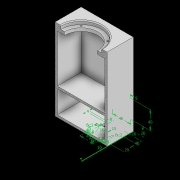
# Autodesk Inventor part: groovev2
Saved by Autodesk Inventor 2022 (Build 260153000, 153)
## iProperties
Created: 2022-06-28
Part Number: groovev2
Material: Generic
Document SubType Name: Modeling
Designer: Fuzzyfish
Density: 1 g/cm^3
Appearance: Default
Author: Fuzzyfish
Autodesk Inventor part; units mm, degrees
ref_plane "YZ Plane" through (0, 0, 0) normal (1, 0, 0) x (0, 1, 0)
ref_plane "XZ Plane" through (0, 0, 0) normal (0, 1, 0) x (-1, 0, 0)
sketch "Sketch1" plane through (0, 0, 0) normal (0, 1, 0) x (-1, 0, 0)
  line L0 (0, 0) -> (105, 0)
  line L1 (105, 0) -> (105, -105)
  line L2 (105, -105) -> (0, -105)
  line L3 (0, -105) -> (0, 0)
  circle A0 centre (52.5, -52.5) radius 36.5
  dimension "d0" = 105
  dimension "d1" = 105
  dimension "d2" = 52.5
  dimension "d3" = 52.5
  dimension "d4" = 73
  constraints: 8 end point, 2 parallel, 1 centre point, 1 horizontal, 1 perpendicular
  measures "d0" distance of L0.end L1.end
  measures "d1" distance of L1.end L2.end
  measures "d2" distance from line of L1 A0.centre
  measures "d3" distance from line of L0 A0.centre
  measures "d4" diameter of A0
extrude "Extrusion1" add sketch "Sketch1" along normal blind 7
sketch "Sketch3" plane through (-105, 0, 0) normal (0, 0, 1) x (1, 0, 0)
  line L0 (105, 7) -> (0, 7) projected
  line L1 (0, 7) -> (105, 7)
  line L2 (105, 7) -> (105, -105)
  line L3 (105, -105) -> (0, -105)
  line L4 (0, -105) -> (0, 7)
  line L5 (0, 0) -> (105, 0) projected
  dimension "d7" = 105
  constraints: 8 end point, 2 parallel, 1 horizontal, 1 perpendicular
  measures "d7" distance between parallel lines of L5 L3
extrude "Extrusion2" add sketch "Sketch3" along normal blind 5
sketch "Sketch4" plane through (-105, 0, -105) normal (-1, 0, 0) x (0, 0, 1)
  line L0 (0, 0) -> (0, 7) projected
  line L1 (0, 7) -> (110, 7)
  line L2 (110, 7) -> (110, -105)
  line L3 (110, -105) -> (0, -105)
  line L4 (0, -105) -> (0, 7)
  point P0 (105, 0)
  constraints: 8 end point, 2 parallel, 1 horizontal, 1 perpendicular
extrude "Extrusion3" add sketch "Sketch4" along normal blind 5
sketch "Sketch6" plane through (0, 0, -105) normal (0, 0, -1) x (-1, 0, 0)
  line L0 (0, 7) -> (110, 7) projected
  line L1 (110, -105) -> (110, 7) projected
  line L2 (0, 7) -> (110, 7)
  line L3 (110, 7) -> (110, -105)
  line L4 (110, -105) -> (0, -105)
  line L5 (0, -105) -> (0, 7)
  point P0 (0, 0)
  constraints: 8 end point, 2 parallel, 1 horizontal, 1 perpendicular
extrude "Extrusion4" add sketch "Sketch6" along normal blind 5
sketch "Sketch7" plane through (0, -105, 0) normal (1, 0, 0) x (0, 0, -1)
  line L0 (-5, 0) -> (-5, 112) projected
  line L1 (105, 0) -> (110, 0) projected
  line L2 (-5, 112) -> (110, 112)
  line L3 (110, 112) -> (110, 0)
  line L4 (110, 0) -> (-5, 0)
  line L5 (-5, 0) -> (-5, 112)
  point P0 (0, 105)
  constraints: 8 end point, 2 parallel, 1 horizontal, 1 perpendicular
extrude "Extrusion5" add sketch "Sketch7" along normal blind 5
sketch "Sketch8" plane through (-110, -105, -110) normal (0, -1, 0) x (1, 0, 0)
  line L0 (0, 115) -> (115, 115) projected
  line L1 (0, 0) -> (115, 0) projected
  line L2 (0, 115) -> (115, 115)
  line L3 (115, 115) -> (115, 0)
  line L4 (115, 0) -> (0, 0)
  line L5 (0, 0) -> (0, 115)
  point P0 (110, 110)
  constraints: 8 end point, 2 parallel, 1 horizontal, 1 perpendicular
extrude "Extrusion6" add sketch "Sketch8" along normal blind 5
sketch "Sketch9" plane through (0, 7, 0) normal (0, 1, 0) x (1, 0, 0)
  line L0 (-110, -5) -> (-110, 110) projected
  line L1 (-110, -5) -> (5, -5) projected
  line L2 (5, 110) -> (5, -5) projected
  line L3 (-110, 110) -> (5, 110) projected
  circle A0 centre (-52.5, 52.5) radius 36.5 projected
  line L4 (-110, -5) -> (-110, 110) projected
  line L5 (-110, 110) -> (5, 110) projected
  line L6 (-110, -5) -> (5, -5)
  line L7 (5, -5) -> (5, 110)
  line L8 (5, 110) -> (-110, 110)
  line L9 (-110, 110) -> (-110, -5)
  circle A1 centre (-52.5, 52.5) radius 45
  dimension "d18" = 90
  constraints: 8 end point, 2 parallel, 1 centre point, 1 coincident, 1 horizontal, 1 perpendicular
  measures "d18" diameter of A1
extrude "Extrusion7" add sketch "Sketch9" along normal blind 8 contours L0 L3 L2 L1
sketch "Sketch10" plane through (-52.5, 7, -52.5) normal (0, 1, 0) x (1, 0, 0)
  line L0 (57.5, -57.5) -> (-57.5, -57.5) construction
  line L1 (57.5, 57.5) -> (57.5, -57.5) construction
  line L2 (-57.5, -57.5) -> (57.5, 57.5) construction
  line L3 (57.5, 57.5) -> (-57.5, 57.5) construction
  line L4 (-57.5, 57.5) -> (57.5, -57.5) construction
  circle A0 centre (0, 0) radius 41.75 construction
  circle A1 centre (-29.5217, -29.5217) radius 1.9
  circle A2 centre (-29.5217, 29.5217) radius 1.9
  circle A3 centre (29.5217, 29.5217) radius 1.9
  circle A4 centre (29.5217, -29.5217) radius 1.9
  line L5 (0, -57.5) -> (0, 57.5) construction
  point P0 (52.5, -52.5)
  dimension "d21" = 3.8
  dimension "d22" = 83.5
  dimension "d23" = 3.8
  dimension "d24" = 3.8
  dimension "d25" = 3.8
  dimension "d26" = 45
  constraints: 8 end point, 5 centre point, 4 point on circle, 4 point on line, 3 midpoint, 2 perpendicular
  measures "d21" diameter of A1
  measures "d22" diameter of A0
  measures "d23" diameter of A2
  measures "d24" diameter of A3
  measures "d25" diameter of A4
  measures "d26" angle of L5 L2
extrude "Extrusion8" cut sketch "Sketch10" against normal blind 5
ref_plane "Work Plane1" through (0, 0, -52.5) normal (0, 0, -1) x (-1, 0, 0)
split "Split2" [suppressed]
chamfer "Chamfer1" distance 2 angle 45 1 edges at (-97.5, 15, -52.5)
sketch "Sketch15" plane through (0, 0, -52.5) normal (0, 0, -1) x (-1, 0, 0)
  line L0 (105, 14) -> (99.9142, 14)
  line L1 (99.9142, 14) -> (98.5, 12.5858)
  line L2 (98.5, 12.5858) -> (98.5, 6)
  line L3 (98.5, 6) -> (90, 6)
  line L4 (90, 6) -> (90, 1)
  line L5 (90, 1) -> (100, 1)
  arc A0 (106, -5) -> (100, 1) centre (100, -5) ccw
  line L6 (106, -5) -> (106, -100)
  arc A1 (100, -106) -> (106, -100) centre (100, -100) ccw
  line L7 (100, -106) -> (5, -106)
  arc A2 (-1, -100) -> (5, -106) centre (5, -100) ccw
  line L8 (-1, -100) -> (-1, -5)
  arc A3 (5, 1) -> (-1, -5) centre (5, -5) ccw
  line L9 (5, 1) -> (15, 1)
  line L10 (15, 1) -> (15, 6)
  line L11 (15, 6) -> (6.5, 6)
  line L12 (6.5, 6) -> (6.5, 12.5858)
  line L13 (6.5, 12.5858) -> (5.0858, 14)
  line L14 (5.0858, 14) -> (0, 14)
  arc A4 (0, 14) -> (-4, 10) centre (0, 10) ccw
  line L15 (-4, 10) -> (-4, -105)
  arc A5 (-4, -105) -> (0, -109) centre (0, -105) ccw
  line L16 (0, -109) -> (105, -109)
  arc A6 (105, -109) -> (109, -105) centre (105, -105) ccw
  line L17 (109, -105) -> (109, 10)
  arc A7 (109, 10) -> (105, 14) centre (105, 10) ccw
  line L18 (89, 0) -> (89, 7) projected
  line L19 (89, 7) -> (97.5, 7) projected
  line L20 (97.5, 7) -> (97.5, 13) projected
  line L21 (97.5, 13) -> (99.5, 15) projected
  line L22 (99.5, 15) -> (110, 15) projected
  line L23 (110, 15) -> (110, -110) projected
  line L24 (110, -110) -> (-5, -110) projected
  line L25 (-5, -110) -> (-5, 15) projected
  line L26 (-5, 15) -> (5.5, 15) projected
  line L27 (5.5, 15) -> (7.5, 13) projected
  line L28 (7.5, 13) -> (7.5, 7) projected
  line L29 (7.5, 7) -> (16, 7) projected
  line L30 (16, 7) -> (16, 0) projected
  line L31 (16, 0) -> (0, 0) projected
  line L32 (0, 0) -> (0, -105) projected
  line L33 (0, -105) -> (105, -105) projected
  line L34 (105, -105) -> (105, 0) projected
  line L35 (105, 0) -> (89, 0) projected
  constraints: 36 end point, 16 point on circle, 8 centre point
extrude "Extrusion11" [suppressed]
sketch "Sketch16" plane through (-110, -110, -110) normal (0, -1, 0) x (1, 0, 0)
  line L0 (10, 57.5) -> (105, 57.5) projected
  line L1 (10, 57.5) -> (10, 54.5) projected
  line L2 (10, 54.5) -> (105, 54.5) projected
  line L3 (105, 57.5) -> (105, 54.5) projected
  circle A0 centre (57.5, 56) radius 2
  line L4 (115, 57.5) -> (0, 57.5) projected
  point P0 (110, 110)
  point P1 (110, 57.5)
  point P2 (5, 57.5)
  dimension "d53" = 95
  dimension "d54" = 47.5
  dimension "d55" = 4
  dimension "d58" = 1.5
  constraints: 1 centre point
  measures "d53" distance of L1.end L2.end
  measures "d54" distance from line of L1 A0.centre
  measures "d55" diameter of A0
  measures "d58" distance from line of L0 A0.centre
extrude "Extrusion14" [suppressed]
sketch "Sketch17" plane through (0, 0, -110) normal (0, 0, -1) x (-1, 0, 0)
  line L0 (110, 15) -> (110, -110) projected
  line L1 (110, -110) -> (-5, -110)
  line L2 (-5, -110) -> (-5, -160)
  line L3 (-5, -160) -> (110, -160)
  line L4 (110, -160) -> (110, -110)
  line L5 (-5, 15) -> (-5, -110) projected
  point P0 (0, 0)
  dimension "d59" = 50
  constraints: 8 end point, 2 parallel, 1 collinear, 1 horizontal, 1 perpendicular
  measures "d59" distance between parallel lines of L1 L3
extrude "Extrusion15" add sketch "Sketch17" against normal blind 5
sketch "Sketch18" plane through (5, -105, 0) normal (1, 0, 0) x (0, 0, -1)
  line L0 (105, -5) -> (-5, -5)
  line L1 (-5, -5) -> (-5, -55)
  line L2 (-5, -55) -> (105, -55)
  line L3 (105, -55) -> (105, -5)
  line L4 (-5, -5) -> (-5, 120) projected
  line L5 (110, -55) -> (105, -55) projected
  point P0 (0, 105)
  constraints: 8 end point, 2 collinear, 2 parallel, 1 horizontal, 1 perpendicular
extrude "Extrusion16" add sketch "Sketch18" against normal blind 5
sketch "Sketch19" plane through (-105, 0, 5) normal (0, 0, 1) x (1, 0, 0)
  line L0 (105, -110) -> (-5, -110) projected
  line L1 (-5, -160) -> (105, -160) projected
  line L2 (-5, -110) -> (105, -110)
  line L3 (105, -110) -> (105, -160)
  line L4 (105, -160) -> (-5, -160)
  line L5 (-5, -160) -> (-5, -110)
  point P0 (105, 0)
  constraints: 8 end point, 2 parallel, 1 horizontal, 1 perpendicular
extrude "Extrusion17" add sketch "Sketch19" against normal blind 5
sketch "Sketch20" plane through (-110, 0, -105) normal (-1, 0, 0) x (0, 0, 1)
  line L0 (-5, -160) -> (110, -160) projected
  line L1 (0, -110) -> (105, -110)
  line L2 (105, -110) -> (105, -160)
  line L3 (105, -160) -> (0, -160)
  line L4 (0, -160) -> (0, -110)
  point P0 (105, 0)
  constraints: 8 end point, 2 parallel, 1 horizontal, 1 perpendicular, 1 point on line
extrude "Extrusion18" add sketch "Sketch20" against normal blind 5
sketch "Sketch21" plane through (-110, -160, -110) normal (0, -1, 0) x (1, 0, 0)
  line L0 (115, 0) -> (0, 0) projected
  line L1 (115, 115) -> (0, 115) projected
  line L2 (0, 0) -> (115, 0)
  line L3 (115, 0) -> (115, 115)
  line L4 (115, 115) -> (0, 115)
  line L5 (0, 115) -> (0, 0)
  point P0 (110, 110)
  constraints: 8 end point, 2 parallel, 1 horizontal, 1 perpendicular
extrude "Extrusion19" add sketch "Sketch21" along normal blind 5
sketch "Sketch25" plane through (-110, -165, -110) normal (0, -1, 0) x (1, 0, 0)
  line L0 (65, 50) -> (105, 50) construction
  line L1 (105, 50) -> (105, 10) construction
  line L2 (105, 10) -> (65, 10) construction
  line L3 (65, 10) -> (65, 50) construction
  line L4 (65, 50) -> (105, 10) construction
  line L5 (105, 50) -> (65, 10) construction
  circle A0 centre (67, 46) radius 1.9
  circle A1 centre (103, 46) radius 1.9
  circle A2 centre (67, 25) radius 1.9
  circle A3 centre (103, 21) radius 1.9
  circle A4 centre (103, 46) radius 3.9
  circle A5 centre (67, 25) radius 3.9
  circle A6 centre (103, 21) radius 3.9
  line L6 (115, 0) -> (115, 115) projected
  line L7 (0, 0) -> (115, 0) projected
  line L8 (83, 14) -> (73, 14)
  line L9 (73, 14) -> (73, 29)
  line L10 (73, 29) -> (83, 29)
  line L11 (83, 29) -> (83, 14)
  line L12 (63, 50) -> (71, 50)
  line L13 (71, 50) -> (71, 42)
  line L14 (71, 42) -> (63, 42)
  line L15 (63, 42) -> (63, 50)
  line L16 (63, 50) -> (71, 42) construction
  line L17 (71, 50) -> (63, 42) construction
  point P0 (110, 110)
  point P1 (85, 30)
  dimension "d101" = 40
  dimension "d102" = 40
  dimension "d103" = 3.8
  dimension "d104" = 3.8
  dimension "d105" = 3.8
  dimension "d106" = 3.8
  dimension "d107" = 4
  dimension "d108" = 2
  dimension "d109" = 2
  dimension "d110" = 4
  dimension "d111" = 25
  dimension "d112" = 2
  dimension "d113" = 29
  dimension "d114" = 2
  dimension "d116" = 2
  dimension "d117" = 2
  dimension "d118" = 2
  dimension "d124" = 10
  dimension "d125" = 10
  dimension "d126" = 10
  dimension "d127" = 15
  dimension "d128" = 4
  dimension "d129" = 8
  dimension "d134" = 4
  dimension "d135" = 4
  dimension "d136" = 8
  dimension "d137" = 8
  constraints: 32 end point, 7 centre point, 6 parallel, 3 coincident, 3 horizontal, 3 perpendicular, 2 midpoint
  measures "d101" distance of L0.start L0.end
  measures "d102" distance of L0.end L1.end
  measures "d103" diameter of A0
  measures "d104" diameter of A1
  measures "d105" diameter of A2
  measures "d106" diameter of A3
  measures "d107" distance from line of L0 A0.centre
  measures "d108" distance from line of L3 A0.centre
  measures "d109" distance from line of L1 A1.centre
  measures "d110" distance from line of L0 A1.centre
  measures "d111" distance from line of L0 A2.centre
  measures "d112" distance from line of L3 A2.centre
  measures "d113" distance from line of L0 A3.centre
  measures "d114" distance from line of L1 A3.centre
  measures "d116" radial gap between concentric circles of A1 A4
  measures "d117" radial gap between concentric circles of A2 A5
  measures "d118" radial gap between concentric circles of A6 A3
  measures "d124" distance between parallel lines of L6 L1
  measures "d125" distance between parallel lines of L7 L2
  measures "d126" distance of L9.end L10.end
  measures "d127" distance of L10.end L8.start
  measures "d128" distance between parallel lines of L8 L2
  measures "d129" distance between parallel lines of L3 L9
  measures "d134" distance from line of A0.centre L13
  measures "d135" distance from line of A0.centre L12
  measures "d136" distance of L12.end L13.end
  measures "d137" distance of L12.start L12.end
extrude "Extrusion23" add sketch "Sketch25" along normal blind 3 contours A4 | A5 | A6
extrude "Extrusion24" cut sketch "Sketch25" along normal blind 3 and the other way blind 5 contours L8 L9 L10 L11
sketch "Sketch26" plane through (0, 0, -110) normal (0, 0, -1) x (-1, 0, 0)
  line L0 (-5, 15) -> (-5, -165) projected
  line L1 (110, -165) -> (-5, -165) projected
  line L2 (105, -160) -> (0, -160) construction
  line L3 (40, -145) -> (0, -145)
  line L4 (0, -145) -> (0, -105)
  line L5 (0, -105) -> (40, -105)
  line L6 (40, -105) -> (40, -145)
  line L7 (33.4662, -145) -> (33.4662, -105) construction
  line L8 (3.4673, -145) -> (3.4673, -105) construction
  line L9 (40, -137.8014) -> (0, -137.8014) construction
  line L10 (0, -160) -> (0, -110) construction
  point P0 (0, 0)
  dimension "d142" = 40
  dimension "d143" = 40
  dimension "d144" = 20
  dimension "d145" = 5
  constraints: 14 end point, 6 point on line, 4 perpendicular, 2 parallel, 1 horizontal
  measures "d142" distance of L3.end L4.end
  measures "d143" distance of L3.start L3.end
  measures "d144" distance between parallel lines of L1 L3
  measures "d145" distance between parallel lines of L0 L4
equation "\"d2\" = 0.5 * d1"
equation "\"d3\" = 0.5 * d0"
equation "\"d23\" = d21"
equation "\"d24\" = d23"
equation "\"d25\" = d24"
equation "\"d54\" = 0.5 * d53"
equation "\"d104\" = d103"
equation "\"d105\" = d103"
equation "\"d106\" = d103"
equation "\"d112\" = d108"
equation "\"d114\" = d109"
equation "\"d116\" = d115"
equation "\"d117\" = d115"
equation "\"d118\" = d115"
equation "\"d115\" = 2"
body "Solid1"
